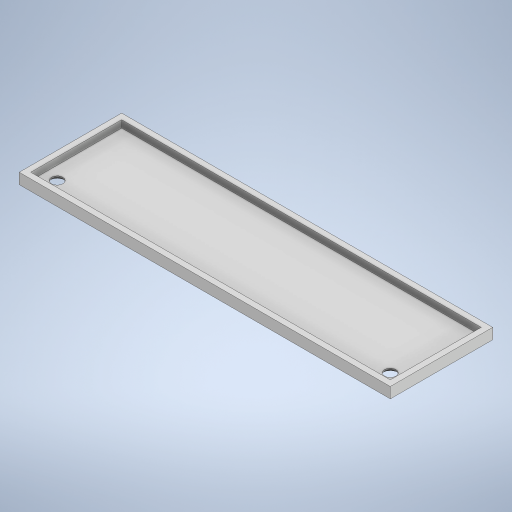
# Autodesk Inventor part: forma_noz
Saved by Autodesk Inventor 2023 (Build 270158000, 158)
## iProperties
Created: 2025-03-20
Part Number: forma_noz
Material: Ogólny
Document SubType Name: Modeling
Designer: kamil
Density: 1 g/cm^3
Appearance: Domyślna
Author: kamil
Autodesk Inventor part; units mm, degrees
ref_plane "YZ Plane" through (0, 0, 0) normal (1, 0, 0) x (0, 1, 0)
ref_plane "XZ Plane" through (0, 0, 0) normal (0, 1, 0) x (-1, 0, 0)
ref_plane "XY Plane" through (0, 0, 0) normal (0, 0, 1) x (1, 0, 0)
sketch "Szkic1" plane through (0, 0, 0) normal (0, 1, 0) x (-1, 0, 0)
  circle A0 centre (3.5, -3.5) radius 1.6
  circle A1 centre (96.5, -3.5) radius 1.6
  line L0 (100, 0) -> (100, -25)
  line L1 (100, -25) -> (0, -25)
  line L2 (0, -25) -> (0, 0)
  line L3 (0, 0) -> (100, 0)
  line L4 (100.2, -25.2) -> (100.2, 0.2)
  line L5 (100.2, 0.2) -> (-0.2, 0.2)
  line L6 (-0.2, 0.2) -> (-0.2, -25.2)
  line L7 (-0.2, -25.2) -> (100.2, -25.2)
  line L8 (101.8, -26.8) -> (101.8, 1.8)
  line L9 (101.8, 1.8) -> (-1.8, 1.8)
  line L10 (-1.8, 1.8) -> (-1.8, -26.8)
  line L11 (-1.8, -26.8) -> (101.8, -26.8)
  dimension "d0" = 0.2
  dimension "d1" = 1.6
  constraints: 24 end point, 2 centre point, 6 other
  measures "d0" distance between parallel lines of L0 L4
  measures "d1" distance between parallel lines of L7 L11
extrude "Wyciągnięcie proste1" add sketch "Szkic1" along normal blind 1 contours L0 L1 L2 L3 | L7 L6 L5 L4 | L11 L10 L9 L8
extrude "Wyciągnięcie proste2" add sketch "Szkic1" along normal blind 3 contours L11 L10 L9 L8
chamfer "Faza1" distance 0.6 angle 45 2 edges at (-1.9, 0, -3.5) (-94.9, 0, -3.5)
